nuxal_reprap4040_Zadjust (Autodesk Fusion 360 design; units mm, degrees)
Autodesk Fusion 360 part; units mm, degrees
sketch "Sketch1" plane through (0, 0, 0) normal (0, 1, 0) x (1, 0, 0)
  line L0 (0, 0) -> (10, 0)
  line L1 (10, 0) -> (10, -10)
  line L2 (10, -10) -> (0, -10)
  line L3 (0, -10) -> (0, 0)
  line L4 (0, -10) -> (10, -10)
  line L5 (10, -10) -> (10, -20)
  line L6 (0, -20) -> (0, -10)
  circle A0 centre (5, -5) radius 1.65
  line L7 (8, -13.5) -> (2, -13.5)
  line L8 (2, -13.5) -> (2, -16.5)
  line L9 (2, -16.5) -> (8, -16.5)
  line L10 (8, -16.5) -> (8, -13.5)
  line L11 (8, -13.5) -> (2, -16.5) construction
  line L12 (2, -13.5) -> (8, -16.5) construction
  line L13 (0, -20) -> (10, -20)
  dimension "d1" = 3.3
  dimension "d2" = 6
  dimension "d3" = 3
  constraint horizontal L0
  constraint vertical L1
  constraint horizontal L2
  constraint vertical L3
  constraint coincident L0.start L3.end
  constraint horizontal L4
  constraint vertical L5
  constraint vertical L6
  constraint perpendicular L7 L8
  constraint parallel L7 L9
  constraint parallel L8 L10
  constraint horizontal L7
  constraint coincident L11
  constraint coincident L12
  measures "d1" diameter of A0
  measures "d3" distance of L0.start
extrude "Extrude1" add sketch "Sketch1" along normal blind 5 contours L0 L1 L2 L3 L4
extrude "Extrude2" add sketch "Sketch1" along normal blind 15 contours L2 L4 L5 L6 L13
sketch "Sketch2" plane through (0, 0, 10) normal (0, 0, -1) x (-1, 0, 0)
  line L0 (-10, 5) -> (0, 5)
  line L1 (0, 5) -> (0, 15)
  line L2 (0, 15) -> (-10, 15)
  line L3 (-10, 15) -> (-10, 5)
  circle A0 centre (-5, 10) radius 1.5
  dimension "d8" = 3
  measures "d8" diameter of A0
extrude "Extrude3" add sketch "Sketch1" along normal blind 15 contours L2 L4 L5 L6 L13 | L7 L8 L9 L10
extrude "Extrude4" cut sketch "Sketch2" against normal blind 20 contours A0
extrude "Extrude5" cut sketch "Sketch1" along normal blind 19 contours L7 L8 L9 L10
